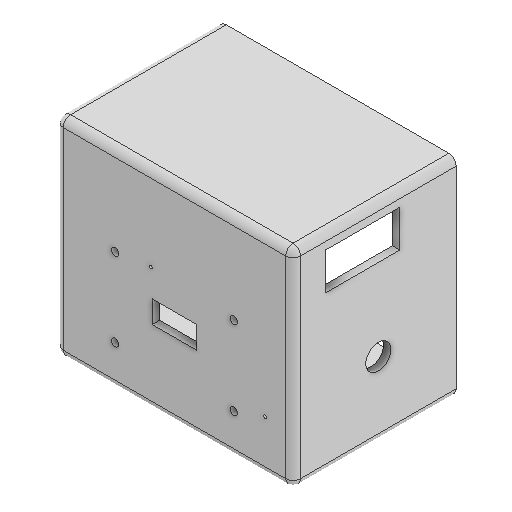
# Autodesk Inventor part: BoxIoT
Saved by Autodesk Inventor 2026.2 (Build 302298010, 298A)
## iProperties
Created: 2026-05-29
Part Number: BoxIoT
Material: Generic
Document SubType Name: Modeling
Designer: rizky
Density: 1 g/cm^3
Appearance: Default
Mass: 404.346 g
Surface Area: 1657.65 cm^2
Volume: 404.346 cm^3
Author: rizky
Autodesk Inventor part; units mm, degrees
ref_plane "YZ Plane" through (0, 0, 0) normal (1, 0, 0) x (0, 1, 0)
ref_plane "XZ Plane" through (0, 0, 0) normal (0, 1, 0) x (-1, 0, 0)
ref_plane "XY Plane" through (0, 0, 0) normal (0, 0, 1) x (1, 0, 0)
sketch "Sketch1" plane through (0, 0, 0) normal (0, 0, 1) x (1, 0, 0)
  line L0 (0, 0) -> (160, 0)
  line L1 (160, 0) -> (160, 140)
  line L2 (160, 140) -> (0, 140)
  line L3 (0, 140) -> (0, 0)
  line L4 (5, 135) -> (155, 135)
  line L5 (155, 135) -> (155, 5)
  line L6 (155, 5) -> (5, 5)
  line L7 (5, 5) -> (5, 135)
  dimension "d0" = 160
  dimension "d1" = 140
  dimension "d2" = 5
  constraints: 16 end point, 4 parallel, 2 perpendicular, 1 horizontal, 3 other
  measures "d0" distance of L2.end L1.end
  measures "d1" distance of L1.end L0.end
  measures "d2" distance between parallel lines of L2 L4
extrude "Extrusion1" add sketch "Sketch1" along normal blind 110
sketch "Sketch2" plane through (0, 0, 110) normal (0, 0, 1) x (1, 0, 0)
  line L0 (160, 0) -> (160, 140) projected
  line L1 (160, 140) -> (0, 140) projected
  line L2 (0, 140) -> (0, 0) projected
  line L3 (0, 0) -> (160, 0) projected
  line L4 (5, 135) -> (155, 135) projected
  line L5 (155, 135) -> (155, 5) projected
  line L6 (155, 5) -> (5, 5) projected
  line L7 (5, 5) -> (5, 135) projected
extrude "Extrusion2" add sketch "Sketch2" against normal blind 5 contours L4 L5 L6 L7
sketch "Sketch4" plane through (160, 0, 0) normal (1, 0, 0) x (0, 0, -1)
  line L0 (0, 0) -> (0, 140) projected
  line L1 (0, 140) -> (-110, 140) projected
  line L2 (-110, 0) -> (-110, 140) projected
  line L3 (0, 0) -> (-110, 0) projected
  line L4 (-110, 140) -> (-110, 130)
  line L5 (-110, 130) -> (-88, 130)
  line L6 (-88, 130) -> (-38, 130)
  line L7 (-38, 130) -> (-38, 105)
  line L8 (-38, 105) -> (-88, 105)
  line L9 (-88, 105) -> (-88, 130)
  point P0 (0, 0)
  dimension "d7" = 10
  dimension "d8" = 22
  dimension "d9" = 50
  dimension "d10" = 25
  constraints: 12 end point, 2 parallel, 2 perpendicular, 1 horizontal, 1 point on line
  measures "d7" distance of L1.end L4.end
  measures "d8" distance of L4.end L5.end
  measures "d9" distance of L7.end L8.end
  measures "d10" distance of L6.end L7.end
extrude "Extrusion3" cut sketch "Sketch4" against normal blind 5 contours L6 L7 L8 L9
sketch "Sketch5" plane through (0, 0, 110) normal (0, 0, 1) x (1, 0, 0)
  line L0 (160, 0) -> (160, 140) projected
  line L1 (160, 140) -> (0, 140) projected
  line L2 (0, 140) -> (0, 0) projected
  line L3 (0, 0) -> (160, 0) projected
  line L4 (80, 140) -> (80, 90)
  line L5 (80, 90) -> (30, 90)
  line L6 (30, 90) -> (30, 17)
  line L7 (30, 17) -> (80, 17)
  line L8 (80, 17) -> (80, 90)
  line L9 (80, 90) -> (130, 90)
  line L10 (130, 90) -> (130, 17)
  line L11 (130, 17) -> (80, 17)
  line L12 (130, 17) -> (120, 17)
  line L13 (120, 17) -> (120, 27)
  circle A0 centre (120, 27) radius 2.5
  line L14 (130, 53.5) -> (125, 53.5)
  circle A1 centre (40, 27) radius 2.5
  circle A2 centre (120, 80) radius 2.5
  circle A3 centre (40, 80) radius 2.5
  dimension "d13" = 50
  dimension "d14" = 50
  dimension "d15" = 73
  dimension "d16" = 10
  dimension "d17" = 10
  dimension "d18" = 5
  dimension "d19" = 5
  constraints: 22 end point, 5 symmetric about line, 4 centre point, 2 horizontal, 2 midpoint, 2 parallel, 2 perpendicular, 1 coincident, 1 point on line, 1 vertical, 3 other
  measures "d13" distance of L4.start L4.end
  measures "d14" distance of L7.end L6.end
  measures "d15" distance of L6.end L5.end
  measures "d16" distance of L11.start L12.end
  measures "d17" distance of L12.end L13.end
  measures "d18" diameter of A0
  measures "d19" distance of L14.start L14.end
extrude "Extrusion4" cut sketch "Sketch5" against normal blind 5 contours A0 | A1 | A2 | A3
sketch "Sketch6" plane through (0, 0, 110) normal (0, 0, 1) x (1, 0, 0)
  circle A0 centre (120, 80) radius 2.5 projected
  circle A1 centre (40, 27) radius 2.5 projected
  circle A2 centre (40, 80) radius 2.5 projected
  circle A3 centre (120, 27) radius 2.5 projected
  line L0 (160, 0) -> (160, 140) projected
  line L1 (160, 140) -> (0, 140) projected
  line L2 (0, 140) -> (0, 0) projected
  line L3 (0, 0) -> (160, 0) projected
  line L4 (160, 0) -> (141.053, 0)
  line L5 (0, 0) -> (160, 0) projected
  line L6 (141.053, 0) -> (141.053, 34.149)
  circle A4 centre (141.053, 34.149) radius 1
  line L7 (0, 140) -> (64.087, 140)
  line L8 (64.087, 140) -> (64.087, 83.191)
  circle A5 centre (64.087, 83.191) radius 1
  dimension "d22" = 18.947
  dimension "d23" = 34.149
  dimension "d24" = 2
  dimension "d28" = 64.087
  dimension "d29" = 56.809
  dimension "d30" = 2
  constraints: 8 end point, 2 centre point, 2 coincident, 2 perpendicular, 2 point on line
  measures "d22" distance of L0.start L4.end
  measures "d23" distance of L4.end L6.end
  measures "d24" diameter of A4
  measures "d28" distance of L1.end L7.end
  measures "d29" distance of L7.end L8.end
  measures "d30" diameter of A5
extrude "Extrusion5" cut sketch "Sketch6" against normal blind 5 contours A4 | A5
fillet "Fillet1" radius 5 8 edges at (160, 0, 55) (0, 0, 55) (160, 140, 55) (0, 140, 55) (80, 0, 110) (0, 70, 110) (80, 140, 110) (160, 70, 110)
sketch "Sketch7" plane through (0, 0, 0) normal (0, 0, -1) x (-1, 0, 0)
  line L0 (-5, 135) -> (-155, 135) projected
  line L1 (-5, 5) -> (-5, 135) projected
  line L2 (-155, 5) -> (-5, 5) projected
  line L3 (-155, 135) -> (-155, 5) projected
  arc A0 (0, 135) -> (-5, 140) centre (-5, 135) ccw projected
  line L4 (-155, 140) -> (-5, 140) projected
  arc A1 (-155, 140) -> (-160, 135) centre (-155, 135) ccw projected
  line L5 (-160, 5) -> (-160, 135) projected
  arc A2 (-160, 5) -> (-155, 0) centre (-155, 5) ccw projected
  line L6 (-5, 0) -> (-155, 0) projected
  arc A3 (-5, 0) -> (0, 5) centre (-5, 5) ccw projected
  line L7 (0, 135) -> (0, 5) projected
  line L8 (-5, 135) -> (-12.5, 135)
  line L9 (-12.5, 135) -> (-12.5, 127.5)
  line L10 (-12.5, 127.5) -> (-5, 127.5)
  line L11 (-5, 127.5) -> (-5, 135)
  circle A4 centre (-12.5, 127.5) radius 1.5
  line L12 (-80, 135) -> (-80, 130)
  line L13 (-5, 70) -> (-10, 70)
  circle A5 centre (-147.5, 127.5) radius 1.5
  circle A6 centre (-12.5, 12.5) radius 1.5
  circle A7 centre (-147.5, 12.5) radius 1.5
  circle A8 centre (-12.5, 127.5) radius 4.5
  line L14 (-5, 123) -> (-12.5, 123)
  line L15 (-5, 5) -> (-5, 135) projected
  line L16 (-17, 127.5) -> (-17, 135)
  circle A9 centre (-147.5, 127.5) radius 4.5
  line L17 (-155, 123) -> (-147.5, 123)
  line L18 (-143, 127.5) -> (-143, 135)
  circle A10 centre (-12.5, 12.5) radius 4.5
  line L19 (-5, 17) -> (-12.5, 17)
  line L20 (-17, 12.5) -> (-17, 5)
  circle A11 centre (-147.5, 12.5) radius 4.5
  line L21 (-143, 12.5) -> (-143, 5)
  line L22 (-155, 17) -> (-147.5, 17)
  point P0 (0, 0)
  dimension "d31" = 7.5
  dimension "d32" = 7.5
  dimension "d33" = 3
  dimension "d34" = 5
  dimension "d35" = 5
  dimension "d36" = 3
  constraints: 28 end point, 18 symmetric about line, 8 centre point, 8 point on circle, 2 horizontal, 2 midpoint, 2 parallel, 2 perpendicular, 2 point on line, 2 tangent, 2 vertical, 1 coincident, 6 other
  measures "d31" distance of L10.end L9.end
  measures "d32" distance of L9.end L8.end
  measures "d33" diameter of A4
  measures "d34" distance of L12.start L12.end
  measures "d35" distance of L13.start L13.end
  measures "d36" radial gap between concentric circles of A4 A8
extrude "Extrusion6" add sketch "Sketch7" against normal blind 10 contours L1 L10 A8 L9 L0 | L9 A8 L16 L0 | L1 L14 A8 L10 | A8 L10 A4 L9 | L9 A4 L10 A8 | L18 A9 L17 L3 L0 | L1 L2 L20 A10 L19 | A9 | A10 | L22 A11 L21 L2 L3 | A11
sketch "Sketch8" plane through (0, 0, 110) normal (0, 0, 1) x (1, 0, 0)
  line L0 (155, 140) -> (5, 140) projected
  line L1 (80, 140) -> (80, 65)
  line L2 (80, 65) -> (65, 65)
  line L3 (65, 65) -> (65, 50)
  line L4 (65, 50) -> (80, 50)
  line L5 (80, 50) -> (80, 65)
  line L6 (80, 65) -> (95, 65)
  line L7 (95, 65) -> (95, 50)
  line L8 (95, 50) -> (80, 50)
  point P0 (0, 0)
  dimension "d39" = 75
  dimension "d40" = 15
  dimension "d41" = 15
  constraints: 16 end point, 2 parallel, 2 symmetric about line, 1 horizontal, 1 midpoint, 1 perpendicular, 1 vertical
  measures "d39" distance of L1.start L1.end
  measures "d40" distance of L4.end L3.end
  measures "d41" distance of L3.end L2.end
extrude "Extrusion7" cut sketch "Sketch8" against normal blind 10
sketch "Sketch9" plane through (160, 5, 0) normal (1, 0, 0) x (0, 0, -1)
  line L0 (0, 135) -> (-105, 135) projected
  line L1 (-110, 130) -> (-110, 0) projected
  line L2 (-105, -5) -> (0, -5) projected
  line L3 (-52.5, 135) -> (-52.5, 45)
  circle A0 centre (-52.5, 45) radius 8.5
  dimension "d44" = 90
  dimension "d45" = 17
  constraints: 2 end point, 1 centre point, 1 coincident, 1 midpoint, 1 vertical
  measures "d44" distance of L3.start L3.end
  measures "d45" diameter of A0
extrude "Extrusion8" cut sketch "Sketch9" against normal blind 10
body "Solid1"
